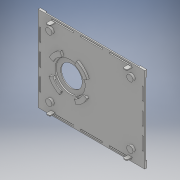
# Autodesk Inventor part: Top Roof
Saved by Autodesk Inventor 2017 (Build 210142000, 142)
## iProperties
Created: 2018-02-08
Part Number: Top Roof
Material: Generic
Document SubType Name: Modeling
Designer: Arjuna
Density: 1 g/cm^3
Appearance: Default
Author: Arjuna
## iProperties of the stored document Top Roof_3DPrint.ipt
Created: 2018-03-30
Part Number: Top Roof_3DPrint
Material: Generic
Document SubType Name: Modeling
Designer: Arjuna
Density: 1 g/cm^3
Appearance: Default
Author: Arjuna
Autodesk Inventor part; units mm, degrees
ref_plane "YZ Plane" through (0, 0, 0) normal (1, 0, 0) x (0, 1, 0)
ref_plane "XZ Plane" through (0, 0, 0) normal (0, 1, 0) x (-1, 0, 0)
ref_plane "XY Plane" through (0, 0, 0) normal (0, 0, 1) x (1, 0, 0)
sketch "Sketch1" plane through (0, 0, 0) normal (0, 1, 0) x (-1, 0, 0)
  line L0 (-125, 100) -> (125, 100)
  line L1 (125, 100) -> (125, -100)
  line L2 (125, -100) -> (-125, -100)
  line L3 (-125, -100) -> (-125, 100)
  point P0 (0, 0)
  dimension "d0" = 200
  dimension "d1" = 250
  dimension "d2" = 125
  dimension "d3" = 100
  constraints: 8 end point, 2 parallel, 1 horizontal, 1 perpendicular
  measures "d0" distance between parallel lines of L2 L0
  measures "d1" distance between parallel lines of L3 L1
  measures "d2" distance from line of point (0, 0) L1
  measures "d3" distance from line of point (0, 0) L0
extrude "Extrusion1" add sketch "Sketch1" along normal blind 5
sketch "Sketch2" plane through (0, 5, 0) normal (0, 1, 0) x (1, 0, 0)
  circle A0 centre (-50, 0) radius 25.25
  point P0 (0, 0)
  dimension "d6" = 50.5
  dimension "d7" = 50
  constraints: 1 centre point
  measures "d6" diameter of A0
  measures "d7" distance of point (0, 0) A0.centre
extrude "Extrusion2" cut sketch "Sketch2" against normal through all
sketch "Sketch3" plane through (0, 0, 0) normal (0, -1, 0) x (1, 0, 0)
  circle A0 centre (-95, -72.5) radius 7.5
  circle A1 centre (-95, 72.5) radius 7.5
  circle A2 centre (95, -72.5) radius 7.5
  circle A3 centre (95, 72.5) radius 7.5
  circle A4 centre (-95, -72.5) radius 8.5
  circle A5 centre (-95, 72.5) radius 8.5
  circle A6 centre (95, 72.5) radius 8.5
  circle A7 centre (95, -72.5) radius 8.5
  point P0 (0, 0)
  dimension "d10" = 15
  dimension "d11" = 72.5
  dimension "d12" = 95
  dimension "d13" = 15
  dimension "d14" = 72.5
  dimension "d15" = 95
  dimension "d16" = 15
  dimension "d17" = 15
  dimension "d18" = 72.5
  dimension "d19" = 72.5
  dimension "d20" = 95
  dimension "d21" = 95
  dimension "d22" = 17
  dimension "d23" = 17
  dimension "d24" = 17
  dimension "d25" = 17
  constraints: 8 centre point, 4 coincident
  measures "d10" diameter of A0
  measures "d11" vertical distance of point (0, 0) A0.centre
  measures "d12" horizontal distance of point (0, 0) A0.centre
  measures "d13" diameter of A1
  measures "d14" vertical distance of point (0, 0) A1.centre
  measures "d15" horizontal distance of point (0, 0) A1.centre
  measures "d16" diameter of A2
  measures "d17" diameter of A3
  measures "d18" vertical distance of point (0, 0) A2.centre
  measures "d19" vertical distance of point (0, 0) A3.centre
  measures "d20" horizontal distance of point (0, 0) A3.centre
  measures "d21" horizontal distance of point (0, 0) A2.centre
  measures "d22" diameter of A4
  measures "d23" diameter of A5
  measures "d24" diameter of A7
  measures "d25" diameter of A6
extrude "Extrusion3" [suppressed]
sketch "Sketch4" plane through (0, 0, 0) normal (0, -1, 0) x (1, 0, 0)
  circle A0 centre (-50, 0) radius 25.25
  circle A1 centre (-50, 0) radius 35.25
  point P0 (0, 0)
  dimension "d28" = 70.5
  dimension "d90" = 50.5
  constraints: 2 centre point, 1 coincident
  measures "d28" diameter of A1
  measures "d90" diameter of A0
extrude "Extrusion4" cut sketch "Sketch4" against normal blind 3
extrude "Extrusion5" add sketch "Sketch3" along normal blind 5 contours A0 | A1 | A2 | A3
sketch "Sketch5" plane through (0, 0, 0) normal (0, -1, 0) x (1, 0, 0)
  line L0 (-115, -92.5) -> (-115, 92.5)
  line L1 (-115, -92.5) -> (115, -92.5)
  line L2 (-115, 92.5) -> (115, 92.5)
  line L3 (115, 92.5) -> (115, -92.5)
  line L4 (-95, -92.5) -> (-85.5, -92.5)
  line L5 (-85.5, -92.5) -> (-85.5, -90.5)
  line L6 (-85.5, -90.5) -> (-95, -90.5)
  line L7 (-95, -90.5) -> (-95, -92.5)
  line L8 (-95, 92.5) -> (-85.5, 92.5)
  line L9 (-85.5, 92.5) -> (-85.5, 90.5)
  line L10 (-85.5, 90.5) -> (-95, 90.5)
  line L11 (-95, 90.5) -> (-95, 92.5)
  line L12 (85.5, -92.5) -> (95, -92.5)
  line L13 (95, -92.5) -> (95, -90.5)
  line L14 (95, -90.5) -> (85.5, -90.5)
  line L15 (85.5, -90.5) -> (85.5, -92.5)
  line L16 (85.5, 92.5) -> (95, 92.5)
  line L17 (95, 92.5) -> (95, 90.5)
  line L18 (95, 90.5) -> (85.5, 90.5)
  line L19 (85.5, 90.5) -> (85.5, 92.5)
  point P0 (0, 0)
  dimension "d33" = 185
  dimension "d34" = 92.5
  dimension "d35" = 230
  dimension "d36" = 115
  dimension "d37" = 9.5
  dimension "d38" = 2
  dimension "d40" = 9.5
  dimension "d41" = 2
  dimension "d43" = 9.5
  dimension "d44" = 2
  dimension "d46" = 2
  dimension "d47" = 9.5
  dimension "d111" = 85.5
  dimension "d112" = 85.5
  dimension "d113" = 85.5
  dimension "d114" = 85.5
  constraints: 40 end point, 8 parallel, 6 horizontal, 5 perpendicular, 4 point on line, 1 vertical
  measures "d33" distance of L0.start L0.end
  measures "d34" vertical distance of point (0, 0) L0.start
  measures "d35" distance of L0.start L1.end
  measures "d36" horizontal distance of point (0, 0) L0.start
  measures "d37" distance of L6.end L5.end
  measures "d38" distance between parallel lines of L6 L1
  measures "d40" distance between parallel lines of L9 L11
  measures "d41" distance between parallel lines of L8 L10
  measures "d43" distance of L14.end L13.end
  measures "d44" distance between parallel lines of L14 L1
  measures "d46" distance between parallel lines of L16 L18
  measures "d47" distance between parallel lines of L17 L19
  measures "d111" distance from line of point (0, 0) L5
  measures "d112" distance from line of point (0, 0) L9
  measures "d113" distance from line of L15 point (0, 0)
  measures "d114" distance from line of point (0, 0) L19
extrude "Extrusion6" add sketch "Sketch5" along normal blind 12 contours L7 L6 L5 L1 | L2 L9 L10 L11 | L15 L14 L13 L1 | L2 L17 L18 L19
chamfer "Chamfer1" distance 2 angle 45 8 edges at (-85.5, -12, -91.5) (-95, -12, -91.5) (-85.5, -12, 91.5) (-95, -12, 91.5) (85.5, -12, 91.5) (95, -12, 91.5) (95, -12, -91.5) (85.5, -12, -91.5)
sketch "Sketch6" plane through (0, 0, 0) normal (0, -1, 0) x (1, 0, 0)
  circle A0 centre (-50, 0) radius 25.25
  circle A1 centre (-50, 0) radius 35.25
  circle A2 centre (-50, 0) radius 43.25
  circle A3 centre (-50, 0) radius 48.5
  point P0 (0, 0)
  dimension "d54" = 86.5
  dimension "d57" = 97
  dimension "d58" = 5.25
  dimension "d91" = 50.5
  dimension "d92" = 70.5
  dimension "d93" = 8
  constraints: 4 centre point, 1 coincident
  measures "d54" diameter of A2
  measures "d57" diameter of A3
  measures "d58" radial gap between concentric circles of A3 A2
  measures "d91" diameter of A0
  measures "d92" diameter of A1
  measures "d93" radial gap between concentric circles of A2 A1
extrude "Extrusion7" add sketch "Sketch6" along normal blind 5 contours A3
sketch "Sketch7" plane through (-50, -5, 0) normal (0, -1, 0) x (1, 0, 0)
  circle A0 centre (0, 0) radius 43.25 projected
  circle A1 centre (0, 0) radius 48.5 projected
  circle A2 centre (0, 0) radius 38.25
  point P0 (50, 0)
  dimension "d61" = 76.5
  dimension "d62" = 5
  constraints: 1 centre point, 1 coincident
  measures "d61" diameter of A2
  measures "d62" radial gap between concentric circles of A0 A2
extrude "Extrusion8" add sketch "Sketch7" against normal blind 2 contours A0
sketch "Sketch8" plane through (-50, -5, 0) normal (0, -1, 0) x (-1, 0, 0)
  circle A0 centre (0, 0) radius 24.5
  circle A1 centre (0, 0) radius 32.5
  line L0 (0, 0) -> (-32.5, 0)
  arc A2 (-30.0261, 12.4372) -> (-32.5, 0) centre (0, 0) ccw
  line L1 (0, 0) -> (-30.0261, 12.4372) construction
  line L2 (0, 0) -> (-32.5, 0) construction
  arc A3 (-32.5, 0) -> (-30.0261, -12.4372) centre (0, 0) ccw
  line L3 (0, 0) -> (-30.0261, -12.4372) construction
  line L4 (0, 0) -> (-32.5, 0) construction
  arc A4 (-22.635, 9.3757) -> (-24.5, 0) centre (0, 0) ccw
  line L5 (0, 0) -> (-22.635, 9.3757) construction
  line L6 (0, 0) -> (-24.5, 0) construction
  arc A5 (-24.5, 0) -> (-22.635, -9.3757) centre (0, 0) ccw
  line L7 (0, 0) -> (-22.635, -9.3757) construction
  line L8 (0, 0) -> (-24.5, 0) construction
  line L9 (-30.0261, -12.4372) -> (-22.635, -9.3757)
  line L10 (-30.0261, 12.4372) -> (-22.635, 9.3757)
  line L11 (-12.4372, -30.0261) -> (-9.3757, -22.635)
  arc A6 (-12.4372, -30.0261) -> (0, -32.5) centre (0, 0) ccw
  arc A7 (0, -24.5) -> (9.3757, -22.635) centre (0, 0) ccw
  line L12 (12.4372, -30.0261) -> (9.3757, -22.635)
  arc A8 (0, -32.5) -> (12.4372, -30.0261) centre (0, 0) ccw
  arc A9 (-9.3757, -22.635) -> (0, -24.5) centre (0, 0) ccw
  line L13 (30.0261, -12.4372) -> (22.635, -9.3757)
  arc A10 (30.0261, -12.4372) -> (32.5, 0) centre (0, 0) ccw
  arc A11 (24.5, 0) -> (22.635, 9.3757) centre (0, 0) ccw
  line L14 (30.0261, 12.4372) -> (22.635, 9.3757)
  arc A12 (32.5, 0) -> (30.0261, 12.4372) centre (0, 0) ccw
  arc A13 (22.635, -9.3757) -> (24.5, 0) centre (0, 0) ccw
  line L15 (12.4372, 30.0261) -> (9.3757, 22.635)
  arc A14 (12.4372, 30.0261) -> (0, 32.5) centre (0, 0) ccw
  arc A15 (0, 24.5) -> (-9.3757, 22.635) centre (0, 0) ccw
  line L16 (-12.4372, 30.0261) -> (-9.3757, 22.635)
  arc A16 (0, 32.5) -> (-12.4372, 30.0261) centre (0, 0) ccw
  arc A17 (9.3757, 22.635) -> (0, 24.5) centre (0, 0) ccw
  point P0 (-50, 0)
  dimension "d65" = 22.5
  dimension "d66" = 22.5
  dimension "d67" = 22.5
  dimension "d68" = 22.5
  dimension "d71" = 360
  constraints: 34 end point, 32 point on circle, 16 centre point, 13 coincident, 2 horizontal alignment, 1 horizontal, 1 point on line, 69 other
  measures "d65" angle of L1 L2
  measures "d66" angle of L4 L3
  measures "d67" angle of L5 L6
  measures "d68" angle of L8 L7
extrude "Extrusion9" [suppressed]
sketch "Sketch9" plane through (-50, -3, 0) normal (0, 1, 0) x (1, 0, 0)
  arc A0 (38.25, 0) -> (38.25, 0) centre (0, 0) ccw projected
  line L0 (6.3338, 15.2912) -> (5.6016, 13.5234) projected
  circle A1 centre (0, 0) radius 48.5 projected
  line L1 (-12.4208, -29.4807) -> (-18.7354, -44.7254)
  line L2 (-12.4208, -29.4807) -> (-18.7354, -44.7254)
  line L3 (-16.5284, -27.6382) -> (-22.8093, -42.8017)
  line L4 (-16.5284, -27.6382) -> (-16.4484, -27.445)
  arc A2 (-16.4484, -27.445) -> (-12.4208, -29.4807) centre (-0.9406, -1.765) ccw
  arc A3 (-22.8093, -42.8017) -> (-18.7354, -44.7254) centre (-0.9406, -1.765) ccw
  circle A4 centre (0, 0) radius 48.5 projected
  circle A5 centre (0, 0) radius 48.5 projected
  circle A6 centre (0, 0) radius 48.5 projected
  line L5 (27.6382, -16.5284) -> (27.445, -16.4484)
  arc A7 (27.445, -16.4484) -> (29.4807, -12.4208) centre (1.765, -0.9406) ccw
  line L6 (27.6382, -16.5284) -> (42.8017, -22.8093)
  line L7 (29.4807, -12.4208) -> (44.7254, -18.7354)
  line L8 (29.4807, -12.4208) -> (44.7254, -18.7354)
  arc A8 (42.8017, -22.8093) -> (44.7254, -18.7354) centre (1.765, -0.9406) ccw
  line L9 (16.5284, 27.6382) -> (16.4484, 27.445)
  arc A9 (16.4484, 27.445) -> (12.4208, 29.4807) centre (0.9406, 1.765) ccw
  line L10 (16.5284, 27.6382) -> (22.8093, 42.8017)
  line L11 (12.4208, 29.4807) -> (18.7354, 44.7254)
  line L12 (12.4208, 29.4807) -> (18.7354, 44.7254)
  arc A10 (22.8093, 42.8017) -> (18.7354, 44.7254) centre (0.9406, 1.765) ccw
  line L13 (-27.6382, 16.5284) -> (-27.445, 16.4484)
  arc A11 (-27.445, 16.4484) -> (-29.4807, 12.4208) centre (-1.765, 0.9406) ccw
  line L14 (-27.6382, 16.5284) -> (-42.8017, 22.8093)
  line L15 (-29.4807, 12.4208) -> (-44.7254, 18.7354)
  line L16 (-29.4807, 12.4208) -> (-44.7254, 18.7354)
  arc A12 (-42.8017, 22.8093) -> (-44.7254, 18.7354) centre (-1.765, 0.9406) ccw
  point P0 (50, 0)
  point P1 (43.25, 0)
  dimension "d80" = 360
  constraints: 32 end point, 16 point on circle, 8 centre point, 4 coincident, 1 collinear, 55 other
extrude "Extrusion10" [suppressed]
sketch "Sketch10" plane through (-50, -3, 0) normal (0, 1, 0) x (1, 0, 0)
  circle A0 centre (0, 0) radius 48.5 projected
  circle A1 centre (0, 0) radius 48.5 projected
  circle A2 centre (0, 0) radius 48.5 projected
  circle A3 centre (0, 0) radius 48.5 projected
  line L0 (-14.6953, -34.4604) -> (-12.796, -29.875)
  arc A4 (-16.2395, -28.1519) -> (-12.796, -29.875) centre (0, 0) ccw
  circle A5 centre (0, 0) radius 43.25 projected
  line L1 (-16.2395, -28.1519) -> (0, 0)
  arc A6 (-18.7064, -32.4284) -> (43.25, 0) centre (1.9845, 3.4403) ccw
  line L2 (-16.2395, -28.1519) -> (-18.7064, -32.4284)
  line L3 (28.1519, -16.2395) -> (32.4829, -18.7379)
  arc A7 (32.4829, -18.7379) -> (0, -35) centre (3.9228, -2.2629) ccw
  arc A8 (28.1519, -16.2395) -> (29.875, -12.796) centre (0, 0) ccw
  line L4 (34.4604, -14.6953) -> (29.875, -12.796)
  line L5 (16.2395, 28.1519) -> (18.7379, 32.4829)
  arc A9 (18.7379, 32.4829) -> (35, 0) centre (2.2629, 3.9228) ccw
  arc A10 (16.2395, 28.1519) -> (12.796, 29.875) centre (0, 0) ccw
  line L6 (14.6953, 34.4604) -> (12.796, 29.875)
  line L7 (-28.1519, 16.2395) -> (-32.4829, 18.7379)
  arc A11 (-32.4829, 18.7379) -> (0, 35) centre (-3.9228, 2.2629) ccw
  arc A12 (-28.1519, 16.2395) -> (-29.875, 12.796) centre (0, 0) ccw
  line L8 (-34.4604, 14.6953) -> (-29.875, 12.796)
  point P0 (50, 0)
  point P1 (-37, 0)
  point P2 (-37, 0)
  constraints: 20 point on circle, 18 end point, 8 centre point, 1 coincident, 1 point on line, 1 other
extrude "Extrusion11" [suppressed]
sketch "Sketch11" plane through (-50, -5, 0) normal (0, -1, 0) x (-1, 0, 0)
  circle A0 centre (0, 0) radius 38.25 projected
  circle A1 centre (0, 0) radius 48.5 projected
  arc A2 (-44.1331, 20.1126) -> (-48.4926, 0.8464) centre (0, 0) ccw
  line L0 (0, 0) -> (-44.1331, 20.1126) construction
  line L1 (0, 0) -> (-48.4926, 0.8464) construction
  arc A3 (-48.4926, 0.8464) -> (-44.8082, -18.5601) centre (0, 0) ccw
  line L2 (0, 0) -> (-44.8082, -18.5601) construction
  line L3 (0, 0) -> (-48.4926, 0.8464) construction
  arc A4 (-34.806, 15.862) -> (-38.2442, 0.6676) centre (0, 0) ccw
  line L4 (0, 0) -> (-34.806, 15.862) construction
  line L5 (0, 0) -> (-38.2442, 0.6676) construction
  arc A5 (-38.2442, 0.6676) -> (-35.3384, -14.6376) centre (0, 0) ccw
  line L6 (0, 0) -> (-35.3384, -14.6376) construction
  line L7 (0, 0) -> (-38.2442, 0.6676) construction
  line L8 (0, 0) -> (-44.8082, -18.5601)
  line L9 (0, 0) -> (-44.1331, 20.1126)
  line L10 (-44.8082, -18.5601) -> (-35.3384, -14.6376)
  line L11 (-34.806, 15.862) -> (-44.1331, 20.1126)
  arc A6 (-15.862, -34.806) -> (-0.6676, -38.2442) centre (0, 0) ccw
  arc A7 (-0.6676, -38.2442) -> (14.6376, -35.3384) centre (0, 0) ccw
  line L12 (18.5601, -44.8082) -> (14.6376, -35.3384)
  arc A8 (-0.8464, -48.4926) -> (18.5601, -44.8082) centre (0, 0) ccw
  line L13 (-15.862, -34.806) -> (-20.1126, -44.1331)
  arc A9 (-20.1126, -44.1331) -> (-0.8464, -48.4926) centre (0, 0) ccw
  arc A10 (34.806, -15.862) -> (38.2442, -0.6676) centre (0, 0) ccw
  arc A11 (38.2442, -0.6676) -> (35.3384, 14.6376) centre (0, 0) ccw
  line L14 (44.8082, 18.5601) -> (35.3384, 14.6376)
  arc A12 (48.4926, -0.8464) -> (44.8082, 18.5601) centre (0, 0) ccw
  line L15 (34.806, -15.862) -> (44.1331, -20.1126)
  arc A13 (44.1331, -20.1126) -> (48.4926, -0.8464) centre (0, 0) ccw
  arc A14 (15.862, 34.806) -> (0.6676, 38.2442) centre (0, 0) ccw
  arc A15 (0.6676, 38.2442) -> (-14.6376, 35.3384) centre (0, 0) ccw
  line L16 (-18.5601, 44.8082) -> (-14.6376, 35.3384)
  arc A16 (0.8464, 48.4926) -> (-18.5601, 44.8082) centre (0, 0) ccw
  line L17 (15.862, 34.806) -> (20.1126, 44.1331)
  arc A17 (20.1126, 44.1331) -> (0.8464, 48.4926) centre (0, 0) ccw
  point P0 (-50, 0)
  dimension "d94" = 23.5
  dimension "d95" = 23.5
  dimension "d96" = 23.5
  dimension "d97" = 23.5
  dimension "d100" = 360
  constraints: 36 end point, 32 point on circle, 16 centre point, 13 coincident, 3 collinear, 69 other
  measures "d94" angle of L0 L1
  measures "d95" angle of L3 L2
  measures "d96" angle of L4 L5
  measures "d97" angle of L7 L6
extrude "Extrusion12" cut sketch "Sketch11" against normal up to surface (5 mm away) contours A0 L14 A1 L15 | A0 L16 A1 L17 | L12 A1 L13 A0 | A0 L8 A1 L9
sketch "Sketch12" plane through (-50, -3, 0) normal (0, 1, 0) x (-1, 0, 0)
  line L0 (-35.3384, 14.6376) -> (-44.8082, 18.5601) projected
  arc A0 (-20.1126, 44.1331) -> (-44.8082, 18.5601) centre (0, 0) ccw projected
  line L1 (-20.1126, 44.1331) -> (-15.862, 34.806) projected
  arc A1 (-15.862, 34.806) -> (-35.3384, 14.6376) centre (0, 0) ccw projected
  arc A2 (-17.9355, 39.3558) -> (-39.9578, 16.5511) centre (0, 0) ccw projected
  arc A3 (-32.6749, 19.885) -> (-35.3384, 14.6376) centre (0, 0) ccw
  arc A4 (-41.4475, 25.1863) -> (-44.8082, 18.5601) centre (0, 0) ccw
  line L2 (-32.6749, 19.885) -> (-41.4475, 25.1863)
  line L3 (-35.3384, 14.6376) -> (-44.8082, 18.5601)
  arc A5 (-25.1863, -41.4475) -> (-18.5601, -44.8082) centre (0, 0) ccw
  line L4 (-19.885, -32.6749) -> (-25.1863, -41.4475)
  line L5 (-14.6376, -35.3384) -> (-18.5601, -44.8082)
  arc A6 (-19.885, -32.6749) -> (-14.6376, -35.3384) centre (0, 0) ccw
  arc A7 (41.4475, -25.1863) -> (44.8082, -18.5601) centre (0, 0) ccw
  line L6 (32.6749, -19.885) -> (41.4475, -25.1863)
  line L7 (35.3384, -14.6376) -> (44.8082, -18.5601)
  arc A8 (32.6749, -19.885) -> (35.3384, -14.6376) centre (0, 0) ccw
  arc A9 (25.1863, 41.4475) -> (18.5601, 44.8082) centre (0, 0) ccw
  line L8 (19.885, 32.6749) -> (25.1863, 41.4475)
  line L9 (14.6376, 35.3384) -> (18.5601, 44.8082)
  arc A10 (19.885, 32.6749) -> (14.6376, 35.3384) centre (0, 0) ccw
  point P0 (-50, 0)
  dimension "d107" = 360
  constraints: 17 point on circle, 16 end point, 8 centre point, 5 coincident, 1 collinear, 1 concentric, 41 other
extrude "Extrusion13" add sketch "Sketch12" along normal up to surface (8 mm away) contours L0 A2 L2 A1 | L0 A0 L2 A2 | L4 A6 L5 A5 | L6 A8 L7 A7 | L8 A10 L9 A9
sketch "Sketch14" plane through (0, 5, 0) normal (0, 1, 0) x (1, 0, 0)
  circle A0 centre (-50, 0) radius 25.25
  line L0 (-125, -100) -> (125, -100)
  line L1 (125, -100) -> (125, 100)
  line L2 (125, 100) -> (-125, 100)
  line L3 (-125, 100) -> (-125, -100)
  line L4 (-110, -100) -> (110, -100)
  line L5 (110, -100) -> (110, -89.5)
  line L6 (110, -89.5) -> (-110, -89.5)
  line L7 (-110, -89.5) -> (-110, -100)
  line L8 (-125, -85) -> (-114.5, -85)
  line L9 (-114.5, -85) -> (-114.5, 85)
  line L10 (-114.5, 85) -> (-125, 85)
  line L11 (-125, 85) -> (-125, -85)
  line L12 (-110, 100) -> (110, 100)
  line L13 (110, 100) -> (110, 89.5)
  line L14 (110, 89.5) -> (-110, 89.5)
  line L15 (-110, 89.5) -> (-110, 100)
  line L16 (125, -85) -> (114.5, -85)
  line L17 (114.5, -85) -> (114.5, 85)
  line L18 (114.5, 85) -> (125, 85)
  line L19 (125, 85) -> (125, -85)
  circle A1 centre (-50, 0) radius 25.25 projected
  line L20 (-125, -100) -> (125, -100) projected
  line L21 (125, -100) -> (125, 100) projected
  line L22 (125, 100) -> (-125, 100) projected
  line L23 (-125, 100) -> (-125, -100) projected
  point P0 (0, 0)
  dimension "d161" = 10.5
  dimension "d162" = 15
  dimension "d163" = 15
  dimension "d164" = 10.5
  dimension "d165" = 15
  dimension "d166" = 15
  dimension "d167" = 10.5
  dimension "d168" = 15
  dimension "d169" = 15
  dimension "d170" = 10.5
  dimension "d171" = 15
  dimension "d172" = 15
  dimension "d173" = 220
  dimension "d174" = 170
  constraints: 40 end point, 8 parallel, 4 horizontal, 4 perpendicular, 4 point on line, 1 centre point
  measures "d161" distance between parallel lines of L6 L0
  measures "d162" distance between parallel lines of L7 L3
  measures "d163" distance between parallel lines of L1 L5
  measures "d164" distance between parallel lines of L9 L3
  measures "d165" distance between parallel lines of L0 L8
  measures "d166" distance between parallel lines of L2 L10
  measures "d167" distance between parallel lines of L2 L14
  measures "d168" distance between parallel lines of L15 L3
  measures "d169" distance between parallel lines of L1 L13
  measures "d170" distance between parallel lines of L1 L17
  measures "d171" distance between parallel lines of L16 L0
  measures "d172" distance between parallel lines of L2 L18
  measures "d173" distance of L4.start L4.end
  measures "d174" distance of L10.end L8.start
extrude "Extrusion15" cut sketch "Sketch14" against normal blind 2.5 contours L7 L6 L5 L0 | L3 L10 L9 L8 | L16 L17 L18 L1 | L2 L13 L14 L15
sketch "Sketch17" plane through (0, 2.5, 0) normal (0, 1, 0) x (1, 0, 0)
  line L0 (125, 85) -> (125, -85) projected
  line L1 (114.5, 85) -> (125, 85) projected
  line L2 (114.5, -85) -> (114.5, 85) projected
  line L3 (125, -85) -> (114.5, -85) projected
  line L4 (118.5, -65.75) -> (121.5, -65.75)
  line L5 (121.5, -65.75) -> (121.5, -34.75)
  line L6 (121.5, -34.75) -> (118.5, -34.75)
  line L7 (118.5, -34.75) -> (118.5, -65.75)
  line L8 (118.5, -15.5) -> (121.5, -15.5)
  line L9 (121.5, -15.5) -> (121.5, 15.5)
  line L10 (121.5, 15.5) -> (118.5, 15.5)
  line L11 (118.5, 15.5) -> (118.5, -15.5)
  line L12 (118.5, 34.75) -> (121.5, 34.75)
  line L13 (121.5, 34.75) -> (121.5, 65.75)
  line L14 (121.5, 65.75) -> (118.5, 65.75)
  line L15 (118.5, 65.75) -> (118.5, 34.75)
  point P0 (0, 0)
  dimension "d223" = 3
  dimension "d224" = 3.5
  dimension "d225" = 10.5
  dimension "d226" = 31
  dimension "d227" = 3
  dimension "d228" = 3
  dimension "d229" = 31
  dimension "d230" = 31
  dimension "d231" = 3.5
  dimension "d232" = 3.5
  dimension "d233" = 170
  dimension "d234" = 19.25
  dimension "d235" = 19.25
  dimension "d236" = 19.25
  dimension "d237" = 19.25
  constraints: 24 end point, 6 parallel, 4 point on line, 3 horizontal, 3 perpendicular
  measures "d223" distance between parallel lines of L5 L7
  measures "d224" distance between parallel lines of L0 L5
  measures "d225" distance of L0.end L2.start
  measures "d226" distance between parallel lines of L6 L4
  measures "d227" distance between parallel lines of L9 L11
  measures "d228" distance between parallel lines of L13 L15
  measures "d229" distance between parallel lines of L10 L8
  measures "d230" distance between parallel lines of L14 L12
  measures "d231" distance between parallel lines of L0 L9
  measures "d232" distance between parallel lines of L0 L13
  measures "d233" distance of L2.start L1.start
  measures "d234" distance between parallel lines of L4 L3
  measures "d235" distance between parallel lines of L8 L6
  measures "d236" distance between parallel lines of L12 L10
  measures "d237" distance between parallel lines of L1 L14
extrude "Extrusion18" cut sketch "Sketch17" against normal through all contours L7 L6 L5 L4 | L11 L10 L9 L8 | L15 L14 L13 L12
mirror "Mirror3" about plane through (0, 0, 0) normal (1, 0, 0) of "Extrusion18"
sketch "Sketch18" plane through (0, 2.5, 0) normal (0, 1, 0) x (1, 0, 0)
  line L0 (-93.25, -93.5) -> (-42.25, -93.5)
  line L1 (-42.25, -93.5) -> (-42.25, -96.5)
  line L2 (-42.25, -96.5) -> (-93.25, -96.5)
  line L3 (-93.25, -96.5) -> (-93.25, -93.5)
  line L4 (-25.5, -93.5) -> (25.5, -93.5)
  line L5 (25.5, -93.5) -> (25.5, -96.5)
  line L6 (25.5, -96.5) -> (-25.5, -96.5)
  line L7 (-25.5, -96.5) -> (-25.5, -93.5)
  line L8 (42.25, -93.5) -> (93.25, -93.5)
  line L9 (93.25, -93.5) -> (93.25, -96.5)
  line L10 (93.25, -96.5) -> (42.25, -96.5)
  line L11 (42.25, -96.5) -> (42.25, -93.5)
  line L12 (110, -100) -> (-110, -100) projected
  line L13 (-110, -100) -> (-110, -89.5) projected
  line L14 (110, -100) -> (-110, -100) projected
  line L15 (110, -89.5) -> (110, -100) projected
  line L16 (-110, -89.5) -> (110, -89.5) projected
  line L17 (-110, -100) -> (-110, -89.5) projected
  point P0 (0, 0)
  dimension "d240" = 3.5
  dimension "d241" = 3
  dimension "d242" = 51
  dimension "d243" = 3
  dimension "d244" = 3
  dimension "d245" = 51
  dimension "d246" = 51
  dimension "d247" = 16.75
  dimension "d248" = 10.5
  dimension "d249" = 220
  dimension "d250" = 16.75
  dimension "d251" = 16.75
  dimension "d252" = 16.75
  constraints: 24 end point, 6 parallel, 4 point on line, 3 horizontal, 3 perpendicular
  measures "d240" distance between parallel lines of L12 L2
  measures "d241" distance between parallel lines of L2 L0
  measures "d242" distance between parallel lines of L1 L3
  measures "d243" distance between parallel lines of L6 L4
  measures "d244" distance between parallel lines of L10 L8
  measures "d245" distance between parallel lines of L5 L7
  measures "d246" distance between parallel lines of L9 L11
  measures "d247" distance between parallel lines of L3 L13
  measures "d248" distance of L12.end L13.end
  measures "d249" distance of L16.start L15.start
  measures "d250" distance between parallel lines of L7 L1
  measures "d251" distance between parallel lines of L11 L5
  measures "d252" distance between parallel lines of L15 L9
extrude "Extrusion19" cut sketch "Sketch18" against normal through all contours L0 L1 L2 L3 | L4 L5 L6 L7 | L8 L9 L10 L11
mirror "Mirror4" about plane through (0, 0, 0) normal (0, 0, 1) of "Extrusion19"
equation "\"d2\" = 0.5 * d1"
equation "\"d3\" = 0.5 * d0"
equation "\"d13\" = d10"
equation "\"d14\" = d11"
equation "\"d15\" = d12"
equation "\"d16\" = d10"
equation "\"d17\" = d10"
equation "\"d18\" = d11"
equation "\"d19\" = d11"
equation "\"d20\" = d12"
equation "\"d21\" = d12"
equation "\"d23\" = d22"
equation "\"d24\" = d22"
equation "\"d25\" = d22"
equation "\"d34\" = 0.5 * d33"
equation "\"d36\" = 0.5 * d35"
equation "\"d40\" = d37"
equation "\"d41\" = d38"
equation "\"d43\" = d37"
equation "\"d44\" = d38"
equation "\"d46\" = d38"
equation "\"d47\" = d37"
equation "\"d112\" = d111"
equation "\"d113\" = d111"
equation "\"d114\" = d111"
equation "\"d94\" = d96"
equation "\"d95\" = d96"
equation "\"d97\" = d96"
equation "\"d163\" = d162"
equation "\"d164\" = d161"
equation "\"d165\" = d162"
equation "\"d166\" = d162"
equation "\"d167\" = d161"
equation "\"d168\" = d162"
equation "\"d169\" = d162"
equation "\"d170\" = d161"
equation "\"d171\" = d162"
equation "\"d172\" = d162"
equation "\"d229\" = d226"
equation "\"d230\" = d226"
equation "\"d234\" = -0.75 * d226 + 0.25 * d233"
equation "\"d235\" = d234"
equation "\"d236\" = d234"
equation "\"d247\" = -0.75 * d242 + 0.25 * d249"
equation "\"d250\" = d247"
equation "\"d251\" = d247"
body "Solid1"
